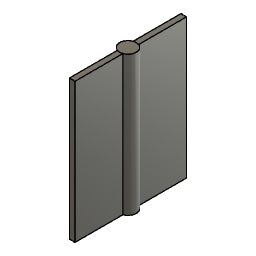
varun (Autodesk Fusion 360 archive; units mm, degrees)
design "arm123"
Autodesk Fusion 360 part; units mm, degrees
(part 1 of 2)
sketch "Sketch1" plane through (0, 0, 0) normal (0, 1, 0) x (1, 0, 0)
  circle A0 centre (0, 0) radius 30
  constraint coincident A0.centre origin
extrude "Extrude1" add sketch "Sketch1" along normal blind 500 makes body 1
sketch "Sketch2" plane through (0, 500, 0) normal (0, 1, 0) x (-1, 0, 0)
  circle A0 centre (0, 0) radius 30
  line L0 (0, 0) -> (10, 0)
  line L1 (10, 0) -> (10, -200)
  line L2 (10, -200) -> (0, -200)
  line L3 (0, 0) -> (-10, 0)
  line L4 (-10, 0) -> (-10, -200)
  line L5 (-10, -200) -> (0, -200)
  constraint horizontal L0
  constraint vertical L1
  constraint horizontal L2
  constraint coincident A0.centre L0.start
  constraint horizontal L3
  constraint vertical L4
  constraint horizontal L5
extrude "Extrude2" add sketch "Sketch2" against normal blind 500 contours A0 L1 L2 L4 L5 bodies 1
pattern_circular "C-Pattern1" count 2 over 360 about axis through (0, 0, 0) along (0, 1, 0) of bodies 1 makes body 2

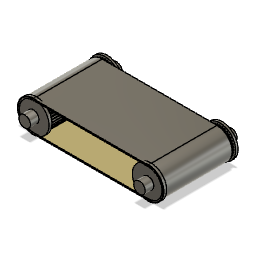
design "conveyer_belt2"
Autodesk Fusion 360 part; units mm, degrees
sketch "Sketch1" plane through (0, 0, 0) normal (0, 0, 1) x (1, 0, 0)
  circle A0 centre (0, 0) radius 221.6972
  constraint coincident A0.centre origin
extrude "Extrude1" add sketch "Sketch1" against normal blind 1200 makes body 1
sketch "Sketch2" plane through (0, 0, 0) normal (0, 0, 1) x (1, 0, 0)
  circle A0 centre (0, 0) radius 221.6972
  line L0 (0, 250.2997) -> (-16.8854, 221.0532)
  line L1 (0, 250.2997) -> (33.7709, 250.2997) construction
  line L2 (0, 250.2997) -> (16.8854, 221.0532)
  line L3 (0, 250.2997) -> (33.6157, 250.2997) construction
  dimension "d3" = 120
  dimension "d4" = 60
  constraint horizontal L1
  constraint horizontal L3
  constraint coincident A0 L0.end
  constraint coincident A0 L2.end
  measures "d3" angle of L0 L1
  measures "d4" angle of L2 L3
extrude "Extrude2" add sketch "Sketch2" against normal blind 1200 contours A0 L0 L2 bodies 1
fillet "Fillet1" radius 4 1 edges at (16.8854, 221.0532, -600) on bodies 1
fillet "Fillet2" radius 4 1 edges at (0, 250.2997, -600) on bodies 1
fillet "Fillet3" radius 4 1 edges at (-16.8854, 221.0532, -600) on bodies 1
pattern_circular "C-Pattern1" count 35 over 360 about axis through (0, 0, 0) along (0, 0, -1) of 5 faces at (7.5882, 237.1566, -800) (16.9768, 221.6146, -800) (2.5712, 245.3638, -400) (-7.5882, 237.1566, -800) (-18.5353, 220.9443, -400) on bodies 1
sketch "Sketch3" plane through (0, 0, 0) normal (0, 0, 1) x (1, 0, 0)
  line L0 (-24.2133, 222.1165) -> (-40.213, 240.9922)
  arc A0 (-40.213, 240.9922) -> (-47.0298, 239.7551) centre (-43.2643, 238.4058) ccw
  line L1 (-47.0298, 239.7551) -> (-55.3768, 216.4612)
  arc A1 (-58.0942, 213.9503) -> (-55.3768, 216.4612) centre (-59.1424, 217.8105) ccw
  arc A2 (-58.0942, 213.9503) -> (-59.8641, 213.4618) centre (0, 0) ccw
  arc A3 (-63.4846, 214.2236) -> (-59.8641, 213.4618) centre (-60.9442, 217.3132) ccw
  line L2 (-63.4846, 214.2236) -> (-82.5975, 229.9391)
  arc A4 (-82.5975, 229.9391) -> (-89.084, 227.5047) centre (-85.138, 226.8494) ccw
  line L3 (-89.084, 227.5047) -> (-93.1375, 203.0946)
  arc A5 (-95.3629, 200.1389) -> (-93.1375, 203.0946) centre (-97.0835, 203.7499) ccw
  arc A6 (-95.3629, 200.1389) -> (-97.0171, 199.3423) centre (0, 0) ccw
  arc A7 (-100.7155, 199.4453) -> (-97.0171, 199.3423) centre (-98.7675, 202.9389) ccw
  line L4 (-100.7155, 199.4453) -> (-122.3274, 211.4955)
  arc A8 (-122.3274, 211.4955) -> (-128.2749, 207.942) centre (-124.2753, 208.0019) ccw
  line L5 (-128.2749, 207.942) -> (-127.9047, 183.2005)
  arc A9 (-129.5665, 179.8949) -> (-127.9047, 183.2005) centre (-131.9043, 183.1406) ccw
  arc A10 (-129.5665, 179.8949) -> (-131.0519, 178.8157) centre (0, 0) ccw
  arc A11 (-134.7093, 178.2567) -> (-131.0519, 178.8157) centre (-133.4164, 182.042) ccw
  line L6 (-134.7093, 178.2567) -> (-158.1255, 186.2543)
  arc A12 (-158.1255, 186.2543) -> (-163.3429, 181.6959) centre (-159.4183, 182.469) ccw
  line L7 (-163.3429, 181.6959) -> (-158.5609, 157.4181)
  arc A13 (-159.6058, 153.8689) -> (-158.5609, 157.4181) centre (-162.4855, 156.6451) ccw
  arc A14 (-159.6058, 153.8689) -> (-160.8746, 152.5418) centre (0, 0) ccw
  arc A15 (-164.3734, 151.3387) -> (-160.8746, 152.5418) centre (-163.7772, 155.2941) ccw
  line L8 (-164.3734, 151.3387) -> (-188.8413, 155.0267)
  arc A16 (-188.8413, 155.0267) -> (-193.161, 149.61) centre (-189.4375, 151.0714) ccw
  line L9 (-193.161, 149.61) -> (-184.1209, 126.5762)
  arc A17 (-184.5152, 122.8974) -> (-184.1209, 126.5762) centre (-187.8444, 125.1148) ccw
  arc A18 (-184.5152, 122.8974) -> (-185.5267, 121.3651) centre (0, 0) ccw
  arc A19 (-188.7544, 119.5567) -> (-185.5267, 121.3651) centre (-188.8741, 123.5549) ccw
  line L10 (-188.7544, 119.5567) -> (-213.4877, 118.8164)
  arc A20 (-213.4877, 118.8164) -> (-216.7707, 112.7155) centre (-213.368, 114.8182) ccw
  line L11 (-216.7707, 112.7155) -> (-203.763, 91.666)
  arc A21 (-203.4942, 87.9759) -> (-203.763, 91.666) centre (-207.1658, 89.5633) ccw
  arc A22 (-203.4942, 87.9759) -> (-204.2158, 86.2877) centre (0, 0) ccw
  arc A23 (-207.0687, 83.9319) -> (-204.2158, 86.2877) centre (-207.9004, 87.8445) ccw
  line L12 (-207.0687, 83.9319) -> (-231.2723, 78.7873)
  arc A24 (-231.2723, 78.7873) -> (-233.4133, 72.1982) centre (-230.4407, 74.8747) ccw
  line L13 (-233.4133, 72.1982) -> (-216.8561, 53.8096)
  arc A25 (-215.9327, 50.2268) -> (-216.8561, 53.8096) centre (-219.8287, 51.1331) ccw
  arc A26 (-215.9327, 50.2268) -> (-216.3412, 48.4369) centre (0, 0) ccw
  arc A27 (-218.7277, 45.6096) -> (-216.3412, 48.4369) centre (-220.2446, 49.3108) ccw
  line L14 (-218.7277, 45.6096) -> (-241.6237, 36.2259)
  arc A28 (-241.6237, 36.2259) -> (-242.5537, 29.3604) centre (-240.1068, 32.5247) ccw
  line L15 (-242.5537, 29.3604) -> (-222.9792, 14.2237)
  arc A29 (-221.4309, 10.8634) -> (-222.9792, 14.2237) centre (-225.4261, 11.0594) ccw
  arc A30 (-221.4309, 10.8634) -> (-221.5133, 9.0292) centre (0, 0) ccw
  arc A31 (-223.3565, 5.8213) -> (-221.5133, 9.0292) centre (-225.51, 9.1921) ccw
  line L16 (-223.3565, 5.8213) -> (-244.2091, -7.4998)
  arc A32 (-244.2091, -7.4998) -> (-243.8983, -14.4211) centre (-242.0557, -10.8707) ccw
  line L17 (-243.8983, -14.4211) -> (-221.9356, -25.8194)
  arc A33 (-219.8121, -28.8492) -> (-221.9356, -25.8194) centre (-223.7781, -29.3697) ccw
  arc A34 (-219.8121, -28.8492) -> (-219.5657, -30.6686) centre (0, 0) ccw
  arc A35 (-220.8065, -34.1541) -> (-219.5657, -30.6686) centre (-223.5272, -31.2219) ccw
  line L18 (-220.8065, -34.1541) -> (-238.9454, -50.9845)
  arc A36 (-238.9454, -50.9845) -> (-237.4037, -57.739) centre (-236.2247, -53.9167) ccw
  line L19 (-237.4037, -57.739) -> (-213.7587, -65.0326)
  arc A37 (-211.1285, -67.6345) -> (-213.7587, -65.0326) centre (-214.9378, -68.8548) ccw
  arc A38 (-211.1285, -67.6345) -> (-210.5611, -69.3807) centre (0, 0) ccw
  arc A39 (-211.1596, -73.0318) -> (-210.5611, -69.3807) centre (-214.3602, -70.6325) ccw
  line L20 (-211.1596, -73.0318) -> (-226.0018, -92.8305)
  arc A40 (-226.0018, -92.8305) -> (-223.2788, -99.2012) centre (-222.8013, -95.2298) ccw
  line L21 (-223.2788, -99.2012) -> (-198.7115, -102.1555)
  arc A41 (-195.6589, -104.2461) -> (-198.7115, -102.1555) centre (-199.1891, -106.1269) ccw
  arc A42 (-195.6589, -104.2461) -> (-194.7889, -105.8629) centre (0, 0) ccw
  arc A43 (-194.7259, -109.5622) -> (-194.7889, -105.8629) centre (-198.3034, -107.7729) ccw
  line L22 (-194.7259, -109.5622) -> (-205.7943, -131.6929)
  arc A44 (-205.7943, -131.6929) -> (-201.9776, -137.475) centre (-202.2168, -133.4822) ccw
  line L23 (-201.9776, -137.475) -> (-177.2776, -135.9952)
  arc A45 (-173.9007, -137.507) -> (-177.2776, -135.9952) centre (-177.0384, -139.988) ccw
  arc A46 (-173.9007, -137.507) -> (-172.756, -138.9425) centre (0, 0) ccw
  arc A47 (-172.0335, -142.5711) -> (-172.756, -138.9425) centre (-175.873, -141.4494) ccw
  line L24 (-172.0335, -142.5711) -> (-178.9725, -166.3225)
  arc A48 (-178.9725, -166.3225) -> (-174.1846, -171.3302) centre (-175.133, -167.4442) ccw
  line L25 (-174.1846, -171.3302) -> (-150.1458, -165.4638)
  arc A49 (-146.5533, -166.3484) -> (-150.1458, -165.4638) centre (-149.1975, -169.3498) ccw
  arc A50 (-146.5533, -166.3484) -> (-145.1706, -167.5564) centre (0, 0) ccw
  arc A51 (-143.8118, -170.9977) -> (-145.1706, -167.5564) centre (-147.7899, -170.5796) ccw
  line L26 (-143.8118, -170.9977) -> (-146.3983, -195.6064)
  arc A52 (-146.3983, -195.6064) -> (-140.7932, -199.6787) centre (-142.4202, -196.0245) ccw
  line L27 (-140.7932, -199.6787) -> (-118.1882, -189.6143)
  arc A53 (-114.4954, -189.8432) -> (-118.1882, -189.6143) centre (-116.5612, -193.2685) ccw
  arc A54 (-114.4954, -189.8432) -> (-112.9193, -190.7849) centre (0, 0) ccw
  arc A55 (-110.9678, -193.9283) -> (-112.9193, -190.7849) centre (-114.9567, -194.2272) ccw
  line L28 (-110.9678, -193.9283) -> (-109.1187, -218.6034)
  arc A56 (-109.1187, -218.6034) -> (-102.8766, -221.6094) centre (-105.1299, -218.3045) ccw
  line L29 (-102.8766, -221.6094) -> (-82.4319, -207.6704)
  arc A57 (-78.7576, -207.2363) -> (-82.4319, -207.6704) centre (-80.1786, -210.9754) ccw
  arc A58 (-78.7576, -207.2363) -> (-77.0387, -207.8815) centre (0, 0) ccw
  arc A59 (-74.5573, -210.6258) -> (-77.0387, -207.8815) centre (-78.4287, -211.6322) ccw
  line L30 (-74.5573, -210.6258) -> (-68.332, -234.5742)
  arc A60 (-68.332, -234.5742) -> (-61.6534, -236.4174) centre (-64.4606, -233.5679) ccw
  line L31 (-61.6534, -236.4174) -> (-44.0262, -219.0519)
  arc A61 (-40.4885, -217.9687) -> (-44.0262, -219.0519) centre (-41.219, -221.9014) ccw
  arc A62 (-40.4885, -217.9687) -> (-38.682, -218.2965) centre (0, 0) ccw
  arc A63 (-35.7505, -220.5537) -> (-38.682, -218.2965) centre (-39.3799, -222.2351) ccw
  line L32 (-35.7505, -220.5537) -> (-25.349, -243.0057)
  arc A64 (-25.349, -243.0057) -> (-18.4487, -243.6267) centre (-21.7196, -241.3242) ccw
  line L33 (-18.4487, -243.6267) -> (-4.2055, -223.3928)
  arc A65 (-0.918, -221.6953) -> (-4.2055, -223.3928) centre (-0.9346, -225.6953) ccw
  arc A66 (-0.918, -221.6953) -> (0.918, -221.6953) centre (0, 0) ccw
  arc A67 (4.2055, -223.3928) -> (0.918, -221.6953) centre (0.9346, -225.6953) ccw
  line L34 (4.2055, -223.3928) -> (18.4487, -243.6267)
  arc A68 (18.4487, -243.6267) -> (25.349, -243.0057) centre (21.7196, -241.3242) ccw
  line L35 (25.349, -243.0057) -> (35.7505, -220.5537)
  arc A69 (38.682, -218.2965) -> (35.7505, -220.5537) centre (39.3799, -222.2351) ccw
  arc A70 (38.682, -218.2965) -> (40.4885, -217.9687) centre (0, 0) ccw
  arc A71 (44.0262, -219.0519) -> (40.4885, -217.9687) centre (41.219, -221.9014) ccw
  line L36 (44.0262, -219.0519) -> (61.6534, -236.4174)
  arc A72 (61.6534, -236.4174) -> (68.332, -234.5742) centre (64.4606, -233.5679) ccw
  line L37 (68.332, -234.5742) -> (74.5573, -210.6258)
  arc A73 (77.0387, -207.8815) -> (74.5573, -210.6258) centre (78.4287, -211.6322) ccw
  arc A74 (77.0387, -207.8815) -> (78.7576, -207.2363) centre (0, 0) ccw
  arc A75 (82.4319, -207.6704) -> (78.7576, -207.2363) centre (80.1786, -210.9754) ccw
  line L38 (82.4319, -207.6704) -> (102.8766, -221.6094)
  arc A76 (102.8766, -221.6094) -> (109.1187, -218.6034) centre (105.1299, -218.3045) ccw
  line L39 (109.1187, -218.6034) -> (110.9678, -193.9283)
  arc A77 (112.9193, -190.7849) -> (110.9678, -193.9283) centre (114.9567, -194.2272) ccw
  arc A78 (112.9193, -190.7849) -> (114.4954, -189.8432) centre (0, 0) ccw
  arc A79 (118.1882, -189.6143) -> (114.4954, -189.8432) centre (116.5612, -193.2685) ccw
  line L40 (118.1882, -189.6143) -> (140.7932, -199.6787)
  arc A80 (140.7932, -199.6787) -> (146.3983, -195.6064) centre (142.4202, -196.0245) ccw
  line L41 (146.3983, -195.6064) -> (143.8118, -170.9977)
  arc A81 (145.1706, -167.5564) -> (143.8118, -170.9977) centre (147.7899, -170.5796) ccw
  arc A82 (145.1706, -167.5564) -> (146.5533, -166.3484) centre (0, 0) ccw
  arc A83 (150.1458, -165.4638) -> (146.5533, -166.3484) centre (149.1975, -169.3498) ccw
  line L42 (150.1458, -165.4638) -> (174.1846, -171.3302)
  arc A84 (174.1846, -171.3302) -> (178.9725, -166.3225) centre (175.133, -167.4442) ccw
  line L43 (178.9725, -166.3225) -> (172.0335, -142.5711)
  arc A85 (172.756, -138.9425) -> (172.0335, -142.5711) centre (175.873, -141.4494) ccw
  arc A86 (172.756, -138.9425) -> (173.9007, -137.507) centre (0, 0) ccw
  arc A87 (177.2776, -135.9952) -> (173.9007, -137.507) centre (177.0384, -139.988) ccw
  line L44 (177.2776, -135.9952) -> (201.9776, -137.475)
  arc A88 (201.9776, -137.475) -> (205.7943, -131.6929) centre (202.2168, -133.4822) ccw
  line L45 (205.7943, -131.6929) -> (194.7259, -109.5622)
  arc A89 (194.7889, -105.8629) -> (194.7259, -109.5622) centre (198.3034, -107.7729) ccw
  arc A90 (194.7889, -105.8629) -> (195.6589, -104.2461) centre (0, 0) ccw
  arc A91 (198.7115, -102.1555) -> (195.6589, -104.2461) centre (199.1891, -106.1269) ccw
  line L46 (198.7115, -102.1555) -> (223.2788, -99.2012)
  arc A92 (223.2788, -99.2012) -> (226.0018, -92.8305) centre (222.8013, -95.2298) ccw
  line L47 (226.0018, -92.8305) -> (211.1596, -73.0318)
  arc A93 (210.5611, -69.3807) -> (211.1596, -73.0318) centre (214.3602, -70.6325) ccw
  arc A94 (210.5611, -69.3807) -> (211.1285, -67.6345) centre (0, 0) ccw
  arc A95 (213.7587, -65.0326) -> (211.1285, -67.6345) centre (214.9378, -68.8548) ccw
  line L48 (213.7587, -65.0326) -> (237.4037, -57.739)
  arc A96 (237.4037, -57.739) -> (238.9454, -50.9845) centre (236.2247, -53.9167) ccw
  line L49 (238.9454, -50.9845) -> (220.8065, -34.1541)
  arc A97 (219.5657, -30.6686) -> (220.8065, -34.1541) centre (223.5272, -31.2219) ccw
  arc A98 (219.5657, -30.6686) -> (219.8121, -28.8492) centre (0, 0) ccw
  arc A99 (221.9356, -25.8194) -> (219.8121, -28.8492) centre (223.7781, -29.3697) ccw
  line L50 (221.9356, -25.8194) -> (243.8983, -14.4211)
  arc A100 (243.8983, -14.4211) -> (244.2091, -7.4998) centre (242.0557, -10.8707) ccw
  line L51 (244.2091, -7.4998) -> (223.3565, 5.8213)
  arc A101 (221.5133, 9.0292) -> (223.3565, 5.8213) centre (225.51, 9.1921) ccw
  arc A102 (221.5133, 9.0292) -> (221.4309, 10.8634) centre (0, 0) ccw
  arc A103 (222.9792, 14.2237) -> (221.4309, 10.8634) centre (225.4261, 11.0594) ccw
  line L52 (222.9792, 14.2237) -> (242.5537, 29.3604)
  arc A104 (242.5537, 29.3604) -> (241.6237, 36.2259) centre (240.1068, 32.5247) ccw
  line L53 (241.6237, 36.2259) -> (218.7277, 45.6096)
  arc A105 (216.3412, 48.4369) -> (218.7277, 45.6096) centre (220.2446, 49.3108) ccw
  arc A106 (216.3412, 48.4369) -> (215.9327, 50.2268) centre (0, 0) ccw
  arc A107 (216.8561, 53.8096) -> (215.9327, 50.2268) centre (219.8287, 51.1331) ccw
  line L54 (216.8561, 53.8096) -> (233.4133, 72.1982)
  arc A108 (233.4133, 72.1982) -> (231.2723, 78.7873) centre (230.4407, 74.8747) ccw
  line L55 (231.2723, 78.7873) -> (207.0687, 83.9319)
  arc A109 (204.2158, 86.2877) -> (207.0687, 83.9319) centre (207.9004, 87.8445) ccw
  arc A110 (204.2158, 86.2877) -> (203.4942, 87.9759) centre (0, 0) ccw
  arc A111 (203.763, 91.666) -> (203.4942, 87.9759) centre (207.1658, 89.5633) ccw
  line L56 (203.763, 91.666) -> (216.7707, 112.7155)
  arc A112 (216.7707, 112.7155) -> (213.4877, 118.8164) centre (213.368, 114.8182) ccw
  line L57 (213.4877, 118.8164) -> (188.7544, 119.5567)
  arc A113 (185.5267, 121.3651) -> (188.7544, 119.5567) centre (188.8741, 123.5549) ccw
  arc A114 (185.5267, 121.3651) -> (184.5152, 122.8974) centre (0, 0) ccw
  arc A115 (184.1209, 126.5762) -> (184.5152, 122.8974) centre (187.8444, 125.1148) ccw
  line L58 (184.1209, 126.5762) -> (193.161, 149.61)
  arc A116 (193.161, 149.61) -> (188.8413, 155.0267) centre (189.4375, 151.0714) ccw
  line L59 (188.8413, 155.0267) -> (164.3734, 151.3387)
  arc A117 (160.8746, 152.5418) -> (164.3734, 151.3387) centre (163.7772, 155.2941) ccw
  arc A118 (160.8746, 152.5418) -> (159.6058, 153.8689) centre (0, 0) ccw
  arc A119 (158.5609, 157.4181) -> (159.6058, 153.8689) centre (162.4855, 156.6451) ccw
  line L60 (158.5609, 157.4181) -> (163.3429, 181.6959)
  arc A120 (163.3429, 181.6959) -> (158.1255, 186.2543) centre (159.4183, 182.469) ccw
  line L61 (158.1255, 186.2543) -> (134.7093, 178.2567)
  arc A121 (131.0519, 178.8157) -> (134.7093, 178.2567) centre (133.4164, 182.042) ccw
  arc A122 (131.0519, 178.8157) -> (129.5665, 179.8949) centre (0, 0) ccw
  arc A123 (127.9047, 183.2005) -> (129.5665, 179.8949) centre (131.9043, 183.1406) ccw
  line L62 (127.9047, 183.2005) -> (128.2749, 207.942)
  arc A124 (128.2749, 207.942) -> (122.3274, 211.4955) centre (124.2753, 208.0019) ccw
  line L63 (122.3274, 211.4955) -> (100.7155, 199.4453)
  arc A125 (97.0171, 199.3423) -> (100.7155, 199.4453) centre (98.7675, 202.9389) ccw
  arc A126 (97.0171, 199.3423) -> (95.3629, 200.1389) centre (0, 0) ccw
  arc A127 (93.1375, 203.0946) -> (95.3629, 200.1389) centre (97.0835, 203.7499) ccw
  line L64 (93.1375, 203.0946) -> (89.084, 227.5047)
  arc A128 (89.084, 227.5047) -> (82.5975, 229.9391) centre (85.138, 226.8494) ccw
  line L65 (82.5975, 229.9391) -> (63.4846, 214.2236)
  arc A129 (59.8641, 213.4618) -> (63.4846, 214.2236) centre (60.9442, 217.3132) ccw
  arc A130 (59.8641, 213.4618) -> (58.0942, 213.9503) centre (0, 0) ccw
  arc A131 (55.3768, 216.4612) -> (58.0942, 213.9503) centre (59.1424, 217.8105) ccw
  line L66 (55.3768, 216.4612) -> (47.0298, 239.7551)
  arc A132 (47.0298, 239.7551) -> (40.213, 240.9922) centre (43.2643, 238.4058) ccw
  line L67 (40.213, 240.9922) -> (24.2133, 222.1165)
  arc A133 (20.7869, 220.7205) -> (24.2133, 222.1165) centre (21.162, 224.7029) ccw
  arc A134 (20.7869, 220.7205) -> (18.9583, 220.8851) centre (0, 0) ccw
  arc A135 (15.8363, 222.8705) -> (18.9583, 220.8851) centre (19.3004, 224.8705) ccw
  line L68 (15.8363, 222.8705) -> (3.4641, 244.2997)
  arc A136 (3.4641, 244.2997) -> (-3.4641, 244.2997) centre (0, 242.2997) ccw
  line L69 (-3.4641, 244.2997) -> (-15.8363, 222.8705)
  arc A137 (-18.9583, 220.8851) -> (-15.8363, 222.8705) centre (-19.3004, 224.8705) ccw
  arc A138 (-18.9583, 220.8851) -> (-20.7869, 220.7205) centre (0, 0) ccw
  arc A139 (-24.2133, 222.1165) -> (-20.7869, 220.7205) centre (-21.162, 224.7029) ccw
  circle A140 centre (0, 0) radius 99.7546
  constraint coincident A2.centre A6.centre
extrude "Extrude3" add sketch "Sketch3" along normal blind 200 contours A140 bodies 1
sketch "Sketch4" plane through (0, 0, -1200) normal (0, 0, -1) x (-1, 0, 0)
  line L0 (55.3768, 216.4612) -> (47.0298, 239.7551)
  arc A0 (47.0298, 239.7551) -> (40.213, 240.9922) centre (43.2643, 238.4058) ccw
  line L1 (40.213, 240.9922) -> (24.2133, 222.1165)
  arc A1 (20.7869, 220.7205) -> (24.2133, 222.1165) centre (21.162, 224.7029) ccw
  arc A2 (20.7869, 220.7205) -> (18.9583, 220.8851) centre (0, 0) ccw
  arc A3 (15.8363, 222.8705) -> (18.9583, 220.8851) centre (19.3004, 224.8705) ccw
  line L2 (15.8363, 222.8705) -> (3.4641, 244.2997)
  arc A4 (3.4641, 244.2997) -> (-3.4641, 244.2997) centre (0, 242.2997) ccw
  line L3 (-3.4641, 244.2997) -> (-15.8363, 222.8705)
  arc A5 (-18.9583, 220.8851) -> (-15.8363, 222.8705) centre (-19.3004, 224.8705) ccw
  arc A6 (-18.9583, 220.8851) -> (-20.7869, 220.7205) centre (0, 0) ccw
  arc A7 (-24.2133, 222.1165) -> (-20.7869, 220.7205) centre (-21.162, 224.7029) ccw
  line L4 (-24.2133, 222.1165) -> (-40.213, 240.9922)
  arc A8 (-40.213, 240.9922) -> (-47.0298, 239.7551) centre (-43.2643, 238.4058) ccw
  line L5 (-47.0298, 239.7551) -> (-55.3768, 216.4612)
  arc A9 (-58.0942, 213.9503) -> (-55.3768, 216.4612) centre (-59.1424, 217.8105) ccw
  arc A10 (-58.0942, 213.9503) -> (-59.8641, 213.4618) centre (0, 0) ccw
  arc A11 (-63.4846, 214.2236) -> (-59.8641, 213.4618) centre (-60.9442, 217.3132) ccw
  line L6 (-63.4846, 214.2236) -> (-82.5975, 229.9391)
  arc A12 (-82.5975, 229.9391) -> (-89.084, 227.5047) centre (-85.138, 226.8494) ccw
  line L7 (-89.084, 227.5047) -> (-93.1375, 203.0946)
  arc A13 (-95.3629, 200.1389) -> (-93.1375, 203.0946) centre (-97.0835, 203.7499) ccw
  arc A14 (-95.3629, 200.1389) -> (-97.0171, 199.3423) centre (0, 0) ccw
  arc A15 (-100.7155, 199.4453) -> (-97.0171, 199.3423) centre (-98.7675, 202.9389) ccw
  line L8 (-100.7155, 199.4453) -> (-122.3274, 211.4955)
  arc A16 (-122.3274, 211.4955) -> (-128.2749, 207.942) centre (-124.2753, 208.0019) ccw
  line L9 (-128.2749, 207.942) -> (-127.9047, 183.2005)
  arc A17 (-129.5665, 179.8949) -> (-127.9047, 183.2005) centre (-131.9043, 183.1406) ccw
  arc A18 (-129.5665, 179.8949) -> (-131.0519, 178.8157) centre (0, 0) ccw
  arc A19 (-134.7093, 178.2567) -> (-131.0519, 178.8157) centre (-133.4164, 182.042) ccw
  line L10 (-134.7093, 178.2567) -> (-158.1255, 186.2543)
  arc A20 (-158.1255, 186.2543) -> (-163.3429, 181.6959) centre (-159.4183, 182.469) ccw
  line L11 (-163.3429, 181.6959) -> (-158.5609, 157.4181)
  arc A21 (-159.6058, 153.8689) -> (-158.5609, 157.4181) centre (-162.4855, 156.6451) ccw
  arc A22 (-159.6058, 153.8689) -> (-160.8746, 152.5418) centre (0, 0) ccw
  arc A23 (-164.3734, 151.3387) -> (-160.8746, 152.5418) centre (-163.7772, 155.2941) ccw
  line L12 (-164.3734, 151.3387) -> (-188.8413, 155.0267)
  arc A24 (-188.8413, 155.0267) -> (-193.161, 149.61) centre (-189.4375, 151.0714) ccw
  line L13 (-193.161, 149.61) -> (-184.1209, 126.5762)
  arc A25 (-184.5152, 122.8974) -> (-184.1209, 126.5762) centre (-187.8444, 125.1148) ccw
  arc A26 (-184.5152, 122.8974) -> (-185.5267, 121.3651) centre (0, 0) ccw
  arc A27 (-188.7544, 119.5567) -> (-185.5267, 121.3651) centre (-188.8741, 123.5549) ccw
  line L14 (-188.7544, 119.5567) -> (-213.4877, 118.8164)
  arc A28 (-213.4877, 118.8164) -> (-216.7707, 112.7155) centre (-213.368, 114.8182) ccw
  line L15 (-216.7707, 112.7155) -> (-203.763, 91.666)
  arc A29 (-203.4942, 87.9759) -> (-203.763, 91.666) centre (-207.1658, 89.5633) ccw
  arc A30 (-203.4942, 87.9759) -> (-204.2158, 86.2877) centre (0, 0) ccw
  arc A31 (-207.0687, 83.9319) -> (-204.2158, 86.2877) centre (-207.9004, 87.8445) ccw
  line L16 (-207.0687, 83.9319) -> (-231.2723, 78.7873)
  arc A32 (-231.2723, 78.7873) -> (-233.4133, 72.1982) centre (-230.4407, 74.8747) ccw
  line L17 (-233.4133, 72.1982) -> (-216.8561, 53.8096)
  arc A33 (-215.9327, 50.2268) -> (-216.8561, 53.8096) centre (-219.8287, 51.1331) ccw
  arc A34 (-215.9327, 50.2268) -> (-216.3412, 48.4369) centre (0, 0) ccw
  arc A35 (-218.7277, 45.6096) -> (-216.3412, 48.4369) centre (-220.2446, 49.3108) ccw
  line L18 (-218.7277, 45.6096) -> (-241.6237, 36.2259)
  arc A36 (-241.6237, 36.2259) -> (-242.5537, 29.3604) centre (-240.1068, 32.5247) ccw
  line L19 (-242.5537, 29.3604) -> (-222.9792, 14.2237)
  arc A37 (-221.4309, 10.8634) -> (-222.9792, 14.2237) centre (-225.4261, 11.0594) ccw
  arc A38 (-221.4309, 10.8634) -> (-221.5133, 9.0292) centre (0, 0) ccw
  arc A39 (-223.3565, 5.8213) -> (-221.5133, 9.0292) centre (-225.51, 9.1921) ccw
  line L20 (-223.3565, 5.8213) -> (-244.2091, -7.4998)
  arc A40 (-244.2091, -7.4998) -> (-243.8983, -14.4211) centre (-242.0557, -10.8707) ccw
  line L21 (-243.8983, -14.4211) -> (-221.9356, -25.8194)
  arc A41 (-219.8121, -28.8492) -> (-221.9356, -25.8194) centre (-223.7781, -29.3697) ccw
  arc A42 (-219.8121, -28.8492) -> (-219.5657, -30.6686) centre (0, 0) ccw
  arc A43 (-220.8065, -34.1541) -> (-219.5657, -30.6686) centre (-223.5272, -31.2219) ccw
  line L22 (-220.8065, -34.1541) -> (-238.9454, -50.9845)
  arc A44 (-238.9454, -50.9845) -> (-237.4037, -57.739) centre (-236.2247, -53.9167) ccw
  line L23 (-237.4037, -57.739) -> (-213.7587, -65.0326)
  arc A45 (-211.1285, -67.6345) -> (-213.7587, -65.0326) centre (-214.9378, -68.8548) ccw
  arc A46 (-211.1285, -67.6345) -> (-210.5611, -69.3807) centre (0, 0) ccw
  arc A47 (-211.1596, -73.0318) -> (-210.5611, -69.3807) centre (-214.3602, -70.6325) ccw
  line L24 (-211.1596, -73.0318) -> (-226.0018, -92.8305)
  arc A48 (-226.0018, -92.8305) -> (-223.2788, -99.2012) centre (-222.8013, -95.2298) ccw
  line L25 (-223.2788, -99.2012) -> (-198.7115, -102.1555)
  arc A49 (-195.6589, -104.2461) -> (-198.7115, -102.1555) centre (-199.1891, -106.1269) ccw
  arc A50 (-195.6589, -104.2461) -> (-194.7889, -105.8629) centre (0, 0) ccw
  arc A51 (-194.7259, -109.5622) -> (-194.7889, -105.8629) centre (-198.3034, -107.7729) ccw
  line L26 (-194.7259, -109.5622) -> (-205.7943, -131.6929)
  arc A52 (-205.7943, -131.6929) -> (-201.9776, -137.475) centre (-202.2168, -133.4822) ccw
  line L27 (-201.9776, -137.475) -> (-177.2776, -135.9952)
  arc A53 (-173.9007, -137.507) -> (-177.2776, -135.9952) centre (-177.0384, -139.988) ccw
  arc A54 (-173.9007, -137.507) -> (-172.756, -138.9425) centre (0, 0) ccw
  arc A55 (-172.0335, -142.5711) -> (-172.756, -138.9425) centre (-175.873, -141.4494) ccw
  line L28 (-172.0335, -142.5711) -> (-178.9725, -166.3225)
  arc A56 (-178.9725, -166.3225) -> (-174.1846, -171.3302) centre (-175.133, -167.4442) ccw
  line L29 (-174.1846, -171.3302) -> (-150.1458, -165.4638)
  arc A57 (-146.5533, -166.3484) -> (-150.1458, -165.4638) centre (-149.1975, -169.3498) ccw
  arc A58 (-146.5533, -166.3484) -> (-145.1706, -167.5564) centre (0, 0) ccw
  arc A59 (-143.8118, -170.9977) -> (-145.1706, -167.5564) centre (-147.7899, -170.5796) ccw
  line L30 (-143.8118, -170.9977) -> (-146.3983, -195.6064)
  arc A60 (-146.3983, -195.6064) -> (-140.7932, -199.6787) centre (-142.4202, -196.0245) ccw
  line L31 (-140.7932, -199.6787) -> (-118.1882, -189.6143)
  arc A61 (-114.4954, -189.8432) -> (-118.1882, -189.6143) centre (-116.5612, -193.2685) ccw
  arc A62 (-114.4954, -189.8432) -> (-112.9193, -190.7849) centre (0, 0) ccw
  arc A63 (-110.9678, -193.9283) -> (-112.9193, -190.7849) centre (-114.9567, -194.2272) ccw
  line L32 (-110.9678, -193.9283) -> (-109.1187, -218.6034)
  arc A64 (-109.1187, -218.6034) -> (-102.8766, -221.6094) centre (-105.1299, -218.3045) ccw
  line L33 (-102.8766, -221.6094) -> (-82.4319, -207.6704)
  arc A65 (-78.7576, -207.2363) -> (-82.4319, -207.6704) centre (-80.1786, -210.9754) ccw
  arc A66 (-78.7576, -207.2363) -> (-77.0387, -207.8815) centre (0, 0) ccw
  arc A67 (-74.5573, -210.6258) -> (-77.0387, -207.8815) centre (-78.4287, -211.6322) ccw
  line L34 (-74.5573, -210.6258) -> (-68.332, -234.5742)
  arc A68 (-68.332, -234.5742) -> (-61.6534, -236.4174) centre (-64.4606, -233.5679) ccw
  line L35 (-61.6534, -236.4174) -> (-44.0262, -219.0519)
  arc A69 (-40.4885, -217.9687) -> (-44.0262, -219.0519) centre (-41.219, -221.9014) ccw
  arc A70 (-40.4885, -217.9687) -> (-38.682, -218.2965) centre (0, 0) ccw
  arc A71 (-35.7505, -220.5537) -> (-38.682, -218.2965) centre (-39.3799, -222.2351) ccw
  line L36 (-35.7505, -220.5537) -> (-25.349, -243.0057)
  arc A72 (-25.349, -243.0057) -> (-18.4487, -243.6267) centre (-21.7196, -241.3242) ccw
  line L37 (-18.4487, -243.6267) -> (-4.2055, -223.3928)
  arc A73 (-0.918, -221.6953) -> (-4.2055, -223.3928) centre (-0.9346, -225.6953) ccw
  arc A74 (-0.918, -221.6953) -> (0.918, -221.6953) centre (0, 0) ccw
  arc A75 (4.2055, -223.3928) -> (0.918, -221.6953) centre (0.9346, -225.6953) ccw
  line L38 (4.2055, -223.3928) -> (18.4487, -243.6267)
  arc A76 (18.4487, -243.6267) -> (25.349, -243.0057) centre (21.7196, -241.3242) ccw
  line L39 (25.349, -243.0057) -> (35.7505, -220.5537)
  arc A77 (38.682, -218.2965) -> (35.7505, -220.5537) centre (39.3799, -222.2351) ccw
  arc A78 (38.682, -218.2965) -> (40.4885, -217.9687) centre (0, 0) ccw
  arc A79 (44.0262, -219.0519) -> (40.4885, -217.9687) centre (41.219, -221.9014) ccw
  line L40 (44.0262, -219.0519) -> (61.6534, -236.4174)
  arc A80 (61.6534, -236.4174) -> (68.332, -234.5742) centre (64.4606, -233.5679) ccw
  line L41 (68.332, -234.5742) -> (74.5573, -210.6258)
  arc A81 (77.0387, -207.8815) -> (74.5573, -210.6258) centre (78.4287, -211.6322) ccw
  arc A82 (77.0387, -207.8815) -> (78.7576, -207.2363) centre (0, 0) ccw
  arc A83 (82.4319, -207.6704) -> (78.7576, -207.2363) centre (80.1786, -210.9754) ccw
  line L42 (82.4319, -207.6704) -> (102.8766, -221.6094)
  arc A84 (102.8766, -221.6094) -> (109.1187, -218.6034) centre (105.1299, -218.3045) ccw
  line L43 (109.1187, -218.6034) -> (110.9678, -193.9283)
  arc A85 (112.9193, -190.7849) -> (110.9678, -193.9283) centre (114.9567, -194.2272) ccw
  arc A86 (112.9193, -190.7849) -> (114.4954, -189.8432) centre (0, 0) ccw
  arc A87 (118.1882, -189.6143) -> (114.4954, -189.8432) centre (116.5612, -193.2685) ccw
  line L44 (118.1882, -189.6143) -> (140.7932, -199.6787)
  arc A88 (140.7932, -199.6787) -> (146.3983, -195.6064) centre (142.4202, -196.0245) ccw
  line L45 (146.3983, -195.6064) -> (143.8118, -170.9977)
  arc A89 (145.1706, -167.5564) -> (143.8118, -170.9977) centre (147.7899, -170.5796) ccw
  arc A90 (145.1706, -167.5564) -> (146.5533, -166.3484) centre (0, 0) ccw
  arc A91 (150.1458, -165.4638) -> (146.5533, -166.3484) centre (149.1975, -169.3498) ccw
  line L46 (150.1458, -165.4638) -> (174.1846, -171.3302)
  arc A92 (174.1846, -171.3302) -> (178.9725, -166.3225) centre (175.133, -167.4442) ccw
  line L47 (178.9725, -166.3225) -> (172.0335, -142.5711)
  arc A93 (172.756, -138.9425) -> (172.0335, -142.5711) centre (175.873, -141.4494) ccw
  arc A94 (172.756, -138.9425) -> (173.9007, -137.507) centre (0, 0) ccw
  arc A95 (177.2776, -135.9952) -> (173.9007, -137.507) centre (177.0384, -139.988) ccw
  line L48 (177.2776, -135.9952) -> (201.9776, -137.475)
  arc A96 (201.9776, -137.475) -> (205.7943, -131.6929) centre (202.2168, -133.4822) ccw
  line L49 (205.7943, -131.6929) -> (194.7259, -109.5622)
  arc A97 (194.7889, -105.8629) -> (194.7259, -109.5622) centre (198.3034, -107.7729) ccw
  arc A98 (194.7889, -105.8629) -> (195.6589, -104.2461) centre (0, 0) ccw
  arc A99 (198.7115, -102.1555) -> (195.6589, -104.2461) centre (199.1891, -106.1269) ccw
  line L50 (198.7115, -102.1555) -> (223.2788, -99.2012)
  arc A100 (223.2788, -99.2012) -> (226.0018, -92.8305) centre (222.8013, -95.2298) ccw
  line L51 (226.0018, -92.8305) -> (211.1596, -73.0318)
  arc A101 (210.5611, -69.3807) -> (211.1596, -73.0318) centre (214.3602, -70.6325) ccw
  arc A102 (210.5611, -69.3807) -> (211.1285, -67.6345) centre (0, 0) ccw
  arc A103 (213.7587, -65.0326) -> (211.1285, -67.6345) centre (214.9378, -68.8548) ccw
  line L52 (213.7587, -65.0326) -> (237.4037, -57.739)
  arc A104 (237.4037, -57.739) -> (238.9454, -50.9845) centre (236.2247, -53.9167) ccw
  line L53 (238.9454, -50.9845) -> (220.8065, -34.1541)
  arc A105 (219.5657, -30.6686) -> (220.8065, -34.1541) centre (223.5272, -31.2219) ccw
  arc A106 (219.5657, -30.6686) -> (219.8121, -28.8492) centre (0, 0) ccw
  arc A107 (221.9356, -25.8194) -> (219.8121, -28.8492) centre (223.7781, -29.3697) ccw
  line L54 (221.9356, -25.8194) -> (243.8983, -14.4211)
  arc A108 (243.8983, -14.4211) -> (244.2091, -7.4998) centre (242.0557, -10.8707) ccw
  line L55 (244.2091, -7.4998) -> (223.3565, 5.8213)
  arc A109 (221.5133, 9.0292) -> (223.3565, 5.8213) centre (225.51, 9.1921) ccw
  arc A110 (221.5133, 9.0292) -> (221.4309, 10.8634) centre (0, 0) ccw
  arc A111 (222.9792, 14.2237) -> (221.4309, 10.8634) centre (225.4261, 11.0594) ccw
  line L56 (222.9792, 14.2237) -> (242.5537, 29.3604)
  arc A112 (242.5537, 29.3604) -> (241.6237, 36.2259) centre (240.1068, 32.5247) ccw
  line L57 (241.6237, 36.2259) -> (218.7277, 45.6096)
  arc A113 (216.3412, 48.4369) -> (218.7277, 45.6096) centre (220.2446, 49.3108) ccw
  arc A114 (216.3412, 48.4369) -> (215.9327, 50.2268) centre (0, 0) ccw
  arc A115 (216.8561, 53.8096) -> (215.9327, 50.2268) centre (219.8287, 51.1331) ccw
  line L58 (216.8561, 53.8096) -> (233.4133, 72.1982)
  arc A116 (233.4133, 72.1982) -> (231.2723, 78.7873) centre (230.4407, 74.8747) ccw
  line L59 (231.2723, 78.7873) -> (207.0687, 83.9319)
  arc A117 (204.2158, 86.2877) -> (207.0687, 83.9319) centre (207.9004, 87.8445) ccw
  arc A118 (204.2158, 86.2877) -> (203.4942, 87.9759) centre (0, 0) ccw
  arc A119 (203.763, 91.666) -> (203.4942, 87.9759) centre (207.1658, 89.5633) ccw
  line L60 (203.763, 91.666) -> (216.7707, 112.7155)
  arc A120 (216.7707, 112.7155) -> (213.4877, 118.8164) centre (213.368, 114.8182) ccw
  line L61 (213.4877, 118.8164) -> (188.7544, 119.5567)
  arc A121 (185.5267, 121.3651) -> (188.7544, 119.5567) centre (188.8741, 123.5549) ccw
  arc A122 (185.5267, 121.3651) -> (184.5152, 122.8974) centre (0, 0) ccw
  arc A123 (184.1209, 126.5762) -> (184.5152, 122.8974) centre (187.8444, 125.1148) ccw
  line L62 (184.1209, 126.5762) -> (193.161, 149.61)
  arc A124 (193.161, 149.61) -> (188.8413, 155.0267) centre (189.4375, 151.0714) ccw
  line L63 (188.8413, 155.0267) -> (164.3734, 151.3387)
  arc A125 (160.8746, 152.5418) -> (164.3734, 151.3387) centre (163.7772, 155.2941) ccw
  arc A126 (160.8746, 152.5418) -> (159.6058, 153.8689) centre (0, 0) ccw
  arc A127 (158.5609, 157.4181) -> (159.6058, 153.8689) centre (162.4855, 156.6451) ccw
  line L64 (158.5609, 157.4181) -> (163.3429, 181.6959)
  arc A128 (163.3429, 181.6959) -> (158.1255, 186.2543) centre (159.4183, 182.469) ccw
  line L65 (158.1255, 186.2543) -> (134.7093, 178.2567)
  arc A129 (131.0519, 178.8157) -> (134.7093, 178.2567) centre (133.4164, 182.042) ccw
  arc A130 (131.0519, 178.8157) -> (129.5665, 179.8949) centre (0, 0) ccw
  arc A131 (127.9047, 183.2005) -> (129.5665, 179.8949) centre (131.9043, 183.1406) ccw
  line L66 (127.9047, 183.2005) -> (128.2749, 207.942)
  arc A132 (128.2749, 207.942) -> (122.3274, 211.4955) centre (124.2753, 208.0019) ccw
  line L67 (122.3274, 211.4955) -> (100.7155, 199.4453)
  arc A133 (97.0171, 199.3423) -> (100.7155, 199.4453) centre (98.7675, 202.9389) ccw
  arc A134 (97.0171, 199.3423) -> (95.3629, 200.1389) centre (0, 0) ccw
  arc A135 (93.1375, 203.0946) -> (95.3629, 200.1389) centre (97.0835, 203.7499) ccw
  line L68 (93.1375, 203.0946) -> (89.084, 227.5047)
  arc A136 (89.084, 227.5047) -> (82.5975, 229.9391) centre (85.138, 226.8494) ccw
  line L69 (82.5975, 229.9391) -> (63.4846, 214.2236)
  arc A137 (59.8641, 213.4618) -> (63.4846, 214.2236) centre (60.9442, 217.3132) ccw
  arc A138 (59.8641, 213.4618) -> (58.0942, 213.9503) centre (0, 0) ccw
  arc A139 (55.3768, 216.4612) -> (58.0942, 213.9503) centre (59.1424, 217.8105) ccw
  circle A140 centre (0, 0) radius 100.098
  constraint coincident A2.centre A6.centre
extrude "Extrude4" add sketch "Sketch4" along normal blind 200 contours A140 bodies 1